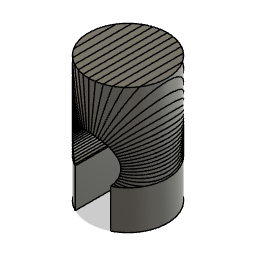
key_hole (Autodesk Fusion 360 design; units mm, degrees)
Autodesk Fusion 360 part; units mm, degrees
note: some values were not read from the file. Chosen so that the rebuilt part matches the saved one: which bodies a step acts on.
sketch "Sketch1" plane through (0, 0, 0) normal (0, 1, 0) x (1, 0, 0)
  circle A0 centre (0, 0) radius 5
  constraint coincident A0.centre origin
extrude "Extrude1" add sketch "Sketch1" against normal blind 7 makes body 1
extrude "Extrude2" add 1 faces at (1.3101, 0, 1.9935) along direction (0, 1, 0) blind 9 on bodies 1 bodies 1
ref_plane "WorkPlane1" through (0, -1.4815, 5) normal (0, 0, 1) x (1, 0, 0)
sketch "Sketch2" plane through (0, 0, 5) normal (0, 0, 1) x (1, 0, 0)
  circle A0 centre (0, 0) radius 3.05
  line L0 (0, 0) -> (-2.25, 0)
  line L1 (-2.25, 0) -> (-2.25, -35)
  line L2 (-2.25, -35) -> (0, -35)
  line L3 (0, -35) -> (0, 0)
  line L4 (0, 0) -> (2.25, 0)
  line L5 (2.25, 0) -> (2.25, -35)
  line L6 (2.25, -35) -> (0, -35)
  line L7 (0, -35) -> (0, 0)
  constraint coincident A0.centre L0.start
  constraint horizontal L0
  constraint vertical L1
  constraint horizontal L2
  constraint vertical L3
  constraint horizontal L4
  constraint vertical L5
  constraint horizontal L6
  constraint vertical L7
  constraint equal L2 L6
extrude "Extrude3" cut sketch "Sketch2" against normal blind 16 bodies 1
ref_plane "WorkPlane2" through (2.25, -2.0591, 4.4651) normal (0, -1, 0) x (1, 0, 0)
split "Split1" by plane through (2.25, -2.0591, 4.4651) normal (0, -1, 0) bodies 1 makes body 2 at (2.25, -3.7061, 1.4884) makes body 3 at (-2.6767, -5.353, 4.2232)
ref_plane "WorkPlane4" through (0, 0, 12.125) normal (0, 1, 0) x (0, 0, 1)
ref_plane "WorkPlane5" through (0, 0, 12.125) normal (-0.087156, 0.996195, 0) x (0, 0, 1)
ref_plane "WorkPlane6" through (0, 0, 12.125) normal (-0.173648, 0.984808, 0) x (0, 0, 1)
ref_plane "WorkPlane7" through (0, 0, 12.125) normal (-0.258819, 0.965926, 0) x (0, 0, 1)
ref_plane "WorkPlane8" through (0, 0, 12.125) normal (-0.34202, 0.939693, 0) x (0, 0, 1)
ref_plane "WorkPlane9" through (0, 0, 12.125) normal (-0.422618, 0.906308, 0) x (0, 0, 1)
ref_plane "WorkPlane10" through (0, 0, 12.125) normal (-0.5, 0.866025, 0) x (0, 0, 1)
ref_plane "WorkPlane11" through (0, 0, 12.125) normal (-0.573576, 0.819152, 0) x (0, 0, 1)
ref_plane "WorkPlane12" through (0, 0, 12.125) normal (-0.642788, 0.766044, 0) x (0, 0, 1)
ref_plane "WorkPlane13" through (0, 0, 12.125) normal (-0.707107, 0.707107, 0) x (0, 0, 1)
ref_plane "WorkPlane14" through (0, 0, 12.125) normal (-0.766044, 0.642788, 0) x (0, 0, 1)
ref_plane "WorkPlane15" through (0, 0, 12.125) normal (-0.819152, 0.573576, 0) x (0, 0, 1)
ref_plane "WorkPlane16" through (0, 0, 12.125) normal (-0.866025, 0.5, 0) x (0, 0, 1)
ref_plane "WorkPlane17" through (0, 0, 12.125) normal (-0.906308, 0.422618, 0) x (0, 0, 1)
ref_plane "WorkPlane18" through (0, 0, 12.125) normal (-0.939693, 0.34202, 0) x (0, 0, 1)
ref_plane "WorkPlane19" through (0, 0, 12.125) normal (-0.965926, 0.258819, 0) x (0, 0, 1)
ref_plane "WorkPlane20" through (0, 0, 12.125) normal (-0.984808, 0.173648, 0) x (0, 0, 1)
ref_plane "WorkPlane21" through (0, 0, 12.125) normal (-0.996195, 0.087156, 0) x (0, 0, 1)
ref_plane "WorkPlane22" through (0, 0, 12.125) normal (-1, 0, 0) x (0, 0, 1)
ref_plane "WorkPlane23" through (0, 0, 12.125) normal (-0.996195, -0.087156, 0) x (0, 0, 1)
ref_plane "WorkPlane24" through (0, 0, 12.125) normal (-0.984808, -0.173648, 0) x (0, 0, 1)
ref_plane "WorkPlane25" through (0, 0, 12.125) normal (-0.965926, -0.258819, 0) x (0, 0, 1)
ref_plane "WorkPlane26" through (0, 0, 12.125) normal (-0.939693, -0.34202, 0) x (0, 0, 1)
ref_plane "WorkPlane27" through (0, 0, 12.125) normal (-0.906308, -0.422618, 0) x (0, 0, 1)
ref_plane "WorkPlane28" through (0, 0, 12.125) normal (-0.866025, -0.5, 0) x (0, 0, 1)
ref_plane "WorkPlane29" through (0, 0, 12.125) normal (-0.819152, -0.573576, 0) x (0, 0, 1)
ref_plane "WorkPlane30" through (0, 0, 12.125) normal (-0.766044, -0.642788, 0) x (0, 0, 1)
ref_plane "WorkPlane31" through (0, 0, 12.125) normal (-0.707107, -0.707107, 0) x (0, 0, 1)
ref_plane "WorkPlane32" through (0, 0, 12.125) normal (-0.642788, -0.766044, 0) x (0, 0, 1)
ref_plane "WorkPlane33" through (0, 0, 12.125) normal (-0.573576, -0.819152, 0) x (0, 0, 1)
ref_plane "WorkPlane34" through (0, 0, 12.125) normal (-0.5, -0.866025, 0) x (0, 0, 1)
ref_plane "WorkPlane35" through (0, 0, 12.125) normal (-0.422618, -0.906308, 0) x (0, 0, 1)
ref_plane "WorkPlane36" through (0, 0, 12.125) normal (-0.34202, -0.939693, 0) x (0, 0, 1)
ref_plane "WorkPlane37" through (0, 0, 12.125) normal (-0.258819, -0.965926, 0) x (0, 0, 1)
ref_plane "WorkPlane38" through (0, 0, 12.125) normal (-0.173648, -0.984808, 0) x (0, 0, 1)
ref_plane "WorkPlane39" through (0, 0, 12.125) normal (-0.087156, -0.996195, 0) x (0, 0, 1)
split "Split2" by plane through (0, 0, 12.125) normal (-0.642788, -0.766044, 0) bodies 1 makes body 4 at (2.318, -2.0591, -1.4521) makes body 5 at (-4.9458, 0.0105, 0.7342)
split "Split3" by plane through (0, 0, 12.125) normal (-0.573576, -0.819152, 0) bodies 1 5 makes body 7 at (-5, -0.2058, 0.0103) makes body 6 at (2.6716, -2.0591, -1.3806)
split "Split4" by plane through (0, 0, 12.125) normal (-0.5, -0.866025, 0) bodies 1 7 makes body 9 at (-3.4322, 0.0333, 3.636) makes body 8 at (3.2221, -2.0591, -1.2242)
split "Split5" by plane through (0, 0, 12.125) normal (-0.422618, -0.906308, 0) bodies 1 9 makes body 11 at (-4.9446, -0.6046, -0.7422) makes body 10 at (2.8771, -1.6611, -1.3756)
split "Split6" by plane through (0, 0, 12.125) normal (-0.34202, -0.939693, 0) bodies 1 11 makes body 13 at (-4.9436, -0.7736, 0.7492) makes body 12 at (3.1126, -1.4514, -1.3507)
split "Split7" by plane through (0, 0, 12.125) normal (-0.258819, -0.965926, 0) bodies 1 13 makes body 15 at (-4.9986, -0.9273, 0.1203) makes body 14 at (3.1727, -1.1548, -1.3071)
split "Split8" by plane through (0, 0, 12.125) normal (-0.173648, -0.984808, 0) bodies 1 15 makes body 17 at (-4.9989, -1.0794, 0.1036) makes body 16 at (3.2769, -0.878, -1.3196)
split "Split9" by plane through (0, 0, 12.125) normal (-0.087156, -0.996195, 0) bodies 1 17 makes body 19 at (-4.932, -1.2299, 0.8219) makes body 18 at (3.3258, -0.5864, -1.3055)
split "Split10" by plane through (0, 0, 12.125) normal (0, 1, 0) bodies 1 19 makes body 21 at (-3.3626, 0.2942, 1.2835) makes body 20 at (-2.6304, 4.5022, 4.2522)
split "Split11" by plane through (0, 0, 12.125) normal (-0.087156, 0.996195, 0) bodies 20 19 makes body 22 at (-3.2252, 0, -1.165) makes body 23 at (-2.6294, 4.5015, 4.2528)
split "Split12" by plane through (0, 0, 12.125) normal (-0.173648, 0.984808, 0) bodies 23 19 makes body 24 at (-3.3626, -0.2942, -1.2835) makes body 25 at (-2.6285, 4.5007, 4.2534)
split "Split13" by plane through (0, 0, 12.125) normal (-0.258819, 0.965926, 0) bodies 25 19 makes body 26 at (-3.3393, -0.5888, -1.3005) makes body 27 at (-2.6275, 4.5, 4.254)
split "Split14" by plane through (0, 0, 12.125) normal (-0.34202, 0.939693, 0) bodies 27 19 makes body 28 at (-3.2836, -0.8798, -1.312) makes body 29 at (-2.6266, 4.4993, 4.2545)
split "Split15" by plane through (0, 0, 12.125) normal (-0.422618, 0.906308, 0) bodies 29 19 makes body 30 at (-3.1718, -1.1544, -1.298) makes body 31 at (-2.6258, 4.4986, 4.255)
split "Split16" by plane through (0, 0, 12.125) normal (-0.5, 0.866025, 0) bodies 31 19 makes body 32 at (-3.1126, -1.4514, -1.3507) makes body 33 at (-2.625, 4.498, 4.2555)
split "Split17" by plane through (0, 0, 12.125) normal (-0.573576, 0.819152, 0) bodies 33 19 makes body 34 at (-2.8771, -1.6611, -1.3756) makes body 35 at (-2.6242, 4.4974, 4.256)
split "Split18" by plane through (0, 0, 12.125) normal (-0.642788, 0.766044, 0) bodies 35 19 makes body 36 at (-2.5362, -1.7759, 1.4212) makes body 37 at (2.6258, 4.4986, 4.255)
split "Split19" by plane through (0, 0, 12.125) normal (-0.707107, 0.707107, 0) bodies 37 makes body 38 at (2.5194, 4.6801, 4.3189)
split "Split20" by plane through (0, 0, 12.125) normal (-0.766044, 0.642788, 0) bodies 38 makes body 39 at (2.4323, 4.8963, 4.3685)
split "Split21" by plane through (0, 0, 12.125) normal (-0.819152, 0.573576, 0) bodies 39 makes body 40 at (2.086, 5.0965, 4.5441)
split "Split22" by plane through (0, 0, 12.125) normal (-0.866025, 0.5, 0) bodies 40 makes body 41 at (1.9533, 5.315, 4.6027)
split "Split23" by plane through (0, 0, 12.125) normal (-0.906308, 0.422618, 0) bodies 41 makes body 42 at (2.8409, 7.1707, 4.1145)
split "Split24" by plane through (0, 0, 12.125) normal (-0.939693, 0.34202, 0) bodies 42 makes body 43 at (1.5039, 5.882, 4.7685)
split "Split25" by plane through (0, 0, 12.125) normal (-0.965926, 0.258819, 0) bodies 43 makes body 44 at (-2.6509, 4.5071, 4.2394)
split "Split26" by plane through (0, 0, 12.125) normal (-0.984808, 0.173648, 0) bodies 44 makes body 45 at (-2.6719, 4.5043, 4.2262)
split "Split27" by plane through (0, 0, 12.125) normal (-0.996195, 0.087156, 0) bodies 45 makes body 46 at (-2.6846, 4.5019, 4.2182)
split "Split28" by plane through (0, 0, 12.125) normal (-1, 0, 0) bodies 46 makes body 47 at (-2.7325, 4.4997, 4.1873)
split "Split29" by plane through (0, 0, 12.125) normal (-0.996195, -0.087156, 0) bodies 47 makes body 48 at (-1.1524, 6.4282, -4.8654)
split "Split30" by plane through (0, 0, 12.125) normal (-0.984808, -0.173648, 0) bodies 48 makes body 49 at (-1.8258, 6.3136, -4.6547)
split "Split31" by plane through (0, 0, 12.125) normal (-0.965926, -0.258819, 0) bodies 49 makes body 50 at (-2.4712, 4.017, 4.3466)
split "Split32" by plane through (0, 0, 12.125) normal (-0.939693, -0.34202, 0) bodies 50 makes body 51 at (-3.0225, 6.2657, -3.983)
split "Split33" by plane through (0, 0, 12.125) normal (-0.906308, -0.422618, 0) bodies 51 makes body 52 at (-2.9624, 5.0121, 4.028)
split "Split34" by plane through (0, 0, 12.125) normal (-0.866025, -0.5, 0) bodies 52 makes body 53 at (-2.9761, 4.2421, 4.0178)
split "Split35" by plane through (0, 0, 12.125) normal (-0.819152, -0.573576, 0) bodies 53 makes body 54 at (-3.051, 3.7477, 3.9613)
split "Split36" by plane through (0, 0, 12.125) normal (-0.766044, -0.642788, 0) bodies 54 makes body 55 at (-2.6621, 2.2338, 1.3678)
split "Split37" by plane through (0, 0, 12.125) normal (-0.707107, -0.707107, 0) bodies 55 makes body 56 at (-2.6621, 2.2338, 1.3678)
move_body "Move1" bodies 24 47 3 46 48 11 36 2 8 55 34 9 43 54 5 56 26 21 39 49 20 40 35 4 19 12 52 6 32 10 28 7 30 25 18 22 13 37 15 50 51 44 14 1 42 17 45 27 33 16 31 53 38 29 23 41 to x (1, 0, 0) y (0, 1, 0) z (0, 0, 1) at (0, 0, -5)
equation "d7 = 2 * 3.05 mm"
